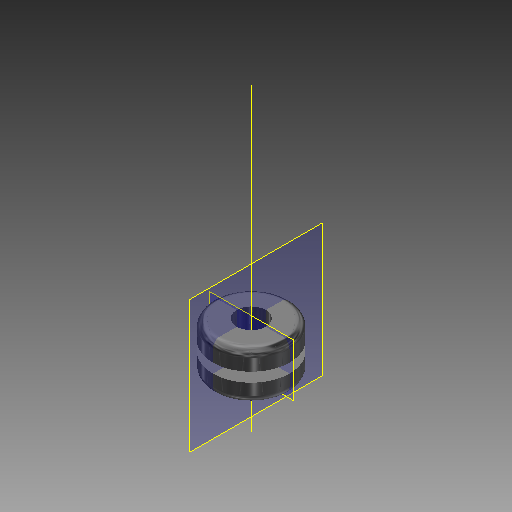
# Autodesk Inventor part: Pneumatic_VIAIAR_00090_05
Saved by Autodesk Inventor 2017 (Build 210142000, 142)
## iProperties
Created: 2011-12-02
Part Number: Pneumatic_VIAIAR_00090_05
Material: Generic
Document SubType Name: Modeling
Designer: Phillip
Density: 1 g/cm^3
Appearance: Rubber - Black - Version 1.1
Author: Phillip
Autodesk Inventor part; units mm, degrees
ref_plane "YZ Plane" through (0, 0, 0) normal (1, 0, 0) x (0, 1, 0)
ref_plane "XZ Plane" through (0, 0, 0) normal (0, 1, 0) x (-1, 0, 0)
ref_plane "XY Plane" through (0, 0, 0) normal (0, 0, 1) x (1, 0, 0)
ref_plane "Work Plane2" through (0.9924, -30.1625, 6.35) normal (-1, 0, 0) x (0, -1, 0)
sketch "Sketch2" plane through (0.9924, -30.1625, 6.35) normal (-1, 0, 0) x (0, -1, 0)
  line L0 (0, -5.5563) -> (0, 3.175) projected
  line L1 (1.5875, -7.1437) -> (1.5875, 3.175) projected
  line L2 (0, 7.1741) -> (-1.905, 7.1741)
  line L3 (-3.175, 5.9041) -> (-3.175, 3.2053)
  arc A0 (-1.905, 7.1741) -> (-3.175, 5.9041) centre (-1.905, 5.9041) ccw
  line L4 (12.0631, 0.7938) -> (-37.2001, 0.7938) projected
  line L5 (-3.175, 3.2053) -> (4.7625, 3.2053)
  line L6 (4.7625, 3.2053) -> (4.7625, 5.9041)
  line L7 (3.4925, 7.1741) -> (1.5875, 7.1741)
  arc A1 (4.7625, 5.9041) -> (3.4925, 7.1741) centre (3.4925, 5.9041) ccw
  line L8 (1.5875, 4.1402) -> (0, 4.1402)
  line L9 (0, 7.1741) -> (0, 4.1402)
  line L10 (1.5875, 7.1741) -> (1.5875, 4.1402)
  point P0 (-30.1625, -6.35)
  point P1 (0, 2.5527)
  point P2 (0, 2.0373)
  point P3 (1.5875, 2.5527)
  dimension "d0" = 1.27
  dimension "d2" = 1.27
  dimension "d4" = 3.9688
  dimension "d5" = 7.9375
  constraints: 16 end point, 4 point on circle, 4 tangent, 3 parallel, 2 centre point, 2 equal length, 2 horizontal, 2 point on line, 2 vertical, 1 perpendicular, 3 other
  measures "d0" radius of A0
  measures "d2" radius of A1
  measures "d4" distance between parallel lines of L5 L2
  measures "d5" distance between parallel lines of L6 L3
revolve "Revolution1" add sketch "Sketch2" angle 360 about axis through (0.9924, -20.447, 7.1438) along (0, 1, 0)
ref_plane "Work Plane3" through (0.9924, -30.9563, 7.1438) normal (0, 0, -1) x (0, -1, 0)
body "Solid1"
